Autodesk Inventor part; units mm, degrees
(part 2 of 3)
  arc A210 (178.5525, 106.028) -> (178.9163, 106.0781) centre (178.3589, 108.7773) ccw projected
  arc A211 (178.9163, 106.0781) -> (180.1512, 106.4453) centre (177.3875, 113.4813) ccw projected
  arc A212 (180.1512, 106.4453) -> (182.401, 107.5925) centre (175.3987, 118.5446) ccw projected
  arc A213 (182.401, 107.5925) -> (182.2553, 109.0714) centre (148.5, 105.0002) ccw projected
  arc A214 (182.2553, 109.0714) -> (179.825, 109.7577) centre (177.5242, 96.9636) ccw projected
  arc A215 (179.825, 109.7577) -> (178.5421, 109.8768) centre (178.487, 102.3176) ccw projected
  arc A216 (178.5421, 109.8768) -> (178.1756, 109.855) centre (178.522, 107.1208) ccw projected
  line L54 (178.1756, 109.855) -> (177.6129, 109.763) projected
  arc A217 (177.6129, 109.763) -> (177.2195, 111.7409) centre (148.5, 105.0002) ccw projected
  line L55 (177.2195, 111.7409) -> (177.7745, 111.8712) projected
  arc A218 (177.7745, 111.8712) -> (178.1215, 111.9914) centre (177.0483, 114.5299) ccw projected
  arc A219 (178.1215, 111.9914) -> (179.2611, 112.5923) centre (175.1778, 118.9541) ccw projected
  arc A220 (179.2611, 112.5923) -> (181.2438, 114.1565) centre (172.2395, 123.5321) ccw projected
  arc A221 (181.2438, 114.1565) -> (180.8125, 115.5785) centre (148.5, 105.0002) ccw projected
  arc A222 (180.8125, 115.5785) -> (178.2949, 115.7775) centre (178.5344, 102.7804) ccw projected
  arc A223 (178.2949, 115.7775) -> (177.0135, 115.644) centre (178.4342, 108.2194) ccw projected
  arc A224 (177.0135, 115.644) -> (176.6582, 115.5512) centre (177.5315, 112.937) ccw projected
  line L56 (176.6582, 115.5512) -> (176.1244, 115.3511) projected
  arc A225 (176.1244, 115.3511) -> (175.3526, 117.2143) centre (148.5, 105.0002) ccw projected
  line L57 (175.3526, 117.2143) -> (175.8716, 117.4504) projected
  arc A226 (175.8716, 117.4504) -> (176.1884, 117.6359) centre (174.6406, 119.9163) ccw projected
  arc A227 (176.1884, 117.6359) -> (177.1889, 118.4477) centre (171.943, 123.8905) ccw projected
  arc A228 (177.1889, 118.4477) -> (178.8284, 120.3685) centre (168.1679, 127.8073) ccw projected
  arc A229 (178.8284, 120.3685) -> (178.1279, 121.6791) centre (148.5, 105.0002) ccw projected
  arc A230 (178.1279, 121.6791) -> (175.6199, 121.3831) centre (178.3903, 108.6825) ccw projected
  arc A231 (175.6199, 121.3831) -> (174.3891, 121.0022) centre (177.231, 113.9974) ccw projected
  arc A232 (174.3891, 121.0022) -> (174.0588, 120.8418) centre (175.4252, 118.4483) ccw projected
  line L58 (174.0588, 120.8418) -> (173.5742, 120.5415) projected
  arc A233 (173.5742, 120.5415) -> (172.4538, 122.2183) centre (148.5, 105.0002) ccw projected
  line L59 (172.4538, 122.2183) -> (172.9167, 122.5511) projected
  arc A234 (172.9167, 122.5511) -> (173.1913, 122.7949) centre (171.2283, 124.7295) ccw projected
  arc A235 (173.1913, 122.7949) -> (174.0142, 123.7862) centre (167.8072, 128.1011) ccw projected
  arc A236 (174.0142, 123.7862) -> (175.2474, 125.99) centre (163.3405, 131.2061) ccw projected
  arc A237 (175.2474, 125.99) -> (174.3047, 127.1387) centre (148.5, 105.0002) ccw projected
  arc A238 (174.3047, 127.1387) -> (171.9026, 126.3591) centre (177.0976, 114.4431) ccw projected
  arc A239 (171.9026, 126.3591) -> (170.7698, 125.7455) centre (174.9236, 119.4296) ccw projected
  arc A240 (170.7698, 125.7455) -> (170.4771, 125.5237) centre (172.2843, 123.4427) ccw projected
  line L60 (170.4771, 125.5237) -> (170.0604, 125.1346) projected
  arc A241 (170.0604, 125.1346) -> (168.6344, 126.5606) centre (148.5, 105.0002) ccw projected
  line L61 (168.6344, 126.5606) -> (169.0235, 126.9773) projected
  arc A242 (169.0235, 126.9773) -> (169.2453, 127.27) centre (166.9426, 128.7845) ccw projected
  arc A243 (169.2453, 127.27) -> (169.8589, 128.4028) centre (162.9294, 131.4238) ccw projected
  arc A244 (169.8589, 128.4028) -> (170.6385, 130.8049) centre (157.9429, 133.5978) ccw projected
  arc A245 (170.6385, 130.8049) -> (169.4898, 131.7476) centre (148.5, 105.0002) ccw projected
  arc A246 (169.4898, 131.7476) -> (167.286, 130.5144) centre (174.7059, 119.8407) ccw projected
  arc A247 (167.286, 130.5144) -> (166.2947, 129.6915) centre (171.6009, 124.3074) ccw projected
  arc A248 (166.2947, 129.6915) -> (166.0509, 129.4169) centre (168.2293, 127.7285) ccw projected
  line L62 (166.0509, 129.4169) -> (165.7181, 128.954) projected
  arc A249 (165.7181, 128.954) -> (164.0413, 130.0744) centre (148.5, 105.0002) ccw projected
  line L63 (164.0413, 130.0744) -> (164.3416, 130.559) projected
  arc A250 (164.3416, 130.559) -> (164.502, 130.8893) centre (161.9481, 131.9254) ccw projected
  arc A251 (164.502, 130.8893) -> (164.8829, 132.1201) centre (157.4972, 133.7312) ccw projected
  arc A252 (164.8829, 132.1201) -> (165.1789, 134.6281) centre (152.1823, 134.8905) ccw projected
  arc A253 (165.1789, 134.6281) -> (163.8683, 135.3286) centre (148.5, 105.0002) ccw projected
  arc A254 (163.8683, 135.3286) -> (161.9475, 133.6891) centre (171.3071, 124.6681) ccw projected
  arc A255 (161.9475, 133.6891) -> (161.1357, 132.6886) centre (167.3903, 128.4432) ccw projected
  circle A256 centre (148.5, 105.0002) radius 2.995
  line L64 (196.9122, 102.2502) -> (196.9122, 107.7502) construction
  line L65 (196.9122, 107.7502) -> (201.6754, 105.0002) construction
  line L66 (201.6754, 105.0002) -> (196.9122, 102.2502) construction
  line L67 (148.5, 105.0002) -> (198.5, 105.0002) construction
  circle A257 centre (201.6754, 105.0002) radius 1.5
  circle A258 centre (196.9122, 102.2502) radius 1.5
  circle A259 centre (196.9122, 107.7502) radius 1.5
  circle A260 centre (198.5, 105.0002) radius 8.5
  line L68 (198.5, 113.5002) -> (157.4972, 113.5002)
  line L69 (198.5, 96.5002) -> (156.0023, 96.5002)
  line L70 (198.5, 105.0002) -> (209.904, 111.5843)
  line L71 (198.5, 105.0002) -> (211.1766, 97.6813)
  line L72 (198.5, 105.0002) -> (198.5, 117.6544)
  line L73 (198.5, 105.0002) -> (198.5, 93.004)
  circle A261 centre (198.5, 105.0002) radius 6
  point P0 (0, 0)
  point P1 (180.5064, 96.5002)
  point P2 (198.5, 99.0002)
  point P3 (203.6961, 102.0002)
  point P4 (205.8612, 100.7502)
  point P5 (205.8612, 109.2502)
  point P6 (203.6961, 108.0002)
  point P7 (198.5, 111.0002)
  point P8 (180.5064, 113.5002)
  dimension "d2" = 5.99
  dimension "d3" = 5.5
  dimension "d4" = 50
  dimension "d5" = 3
  dimension "d6" = 3
  dimension "d7" = 3
  dimension "d8" = 17
  dimension "d9" = 60
  dimension "d10" = 60
  dimension "d11" = 12
  constraints: 20 end point, 6 centre point, 6 coincident, 3 horizontal, 2 point on circle, 2 tangent, 1 collinear, 1 point on line, 1 vertical, 7 other
  measures "d2" diameter of A256
  measures "d3" distance of L64.end L65.end
  measures "d4" distance of L67.start L67.end
  measures "d5" diameter of A257
  measures "d6" diameter of A258
  measures "d7" diameter of A259
  measures "d8" diameter of A260
  measures "d9" angle of L70 L72
  measures "d10" angle of L73 L71
  measures "d11" diameter of A261
extrude "押し出し2" add sketch "スケッチ2" against normal blind 6 contours L68 A260 L69 A198 A199 A200 L50 A201 L51 A202 A203 A204 A205 A206 A207 A208 L52 A209 L53 A210 A211 A212 A213 A214 A215 A216 L54 A217 L55 A218 A219 A220 | L72 A261 L73 A260 | A260 L71 A261 L70 | A261 L70 L72 | L72 L73 A261 | L73 L71 A261 | A261 L71 L70
fillet "フィレット1" radius 2 4 edges at (198.5, 111.0002, 3) (203.6961, 108.0002, 3) (203.6961, 102.0002, 3) (198.5, 99.0002, 3)
extrude "押し出し3" cut sketch "スケッチ2" against normal blind 6 contours A256
sketch "スケッチ3" plane through (0, 0, 6) normal (0, 0, 1) x (1, 0, 0)
  circle A0 centre (148.5, 105.0002) radius 2.995 projected
  circle A1 centre (201.6754, 105.0002) radius 1.5 projected
  circle A2 centre (196.9122, 107.7502) radius 1.5 projected
  circle A3 centre (196.9122, 102.2502) radius 1.5 projected
  arc A4 (161.1357, 132.6886) -> (160.9502, 132.3718) centre (163.4161, 131.1408) ccw projected
  line L0 (160.9502, 132.3718) -> (160.7141, 131.8528) projected
  arc A5 (160.7141, 131.8528) -> (158.8509, 132.6246) centre (148.5, 105.0002) ccw projected
  line L1 (158.8509, 132.6246) -> (159.051, 133.1584) projected
  arc A6 (159.051, 133.1584) -> (159.1439, 133.5137) centre (156.4368, 134.0317) ccw projected
  arc A7 (159.1439, 133.5137) -> (159.2773, 134.7951) centre (151.7192, 134.9344) ccw projected
  arc A8 (159.2773, 134.7951) -> (159.0783, 137.3127) centre (146.2802, 135.0346) ccw projected
  arc A9 (159.0783, 137.3127) -> (157.6563, 137.744) centre (148.5, 105.0002) ccw projected
  arc A10 (157.6563, 137.744) -> (156.0922, 135.7613) centre (167.0319, 128.7396) ccw projected
  arc A11 (156.0922, 135.7613) -> (155.4912, 134.6217) centre (162.4539, 131.678) ccw projected
  arc A12 (155.4912, 134.6217) -> (155.371, 134.2747) centre (158.0297, 133.5485) ccw projected
  line L2 (155.371, 134.2747) -> (155.2407, 133.7197) projected
  arc A13 (155.2407, 133.7197) -> (153.2628, 134.1131) centre (148.5, 105.0002) ccw projected
  line L3 (153.2628, 134.1131) -> (153.3548, 134.6758) projected
  arc A14 (153.3548, 134.6758) -> (153.3766, 135.0423) centre (150.6206, 135.0222) ccw projected
  arc A15 (153.3766, 135.0423) -> (153.2575, 136.3252) centre (145.8174, 134.9872) ccw projected
  arc A16 (153.2575, 136.3252) -> (152.5712, 138.7555) centre (140.4634, 134.0244) ccw projected
  arc A17 (152.5712, 138.7555) -> (151.0923, 138.9012) centre (148.5, 105.0002) ccw projected
  arc A18 (151.0923, 138.9012) -> (149.9451, 136.6514) centre (162.0444, 131.8989) ccw projected
  arc A19 (149.9451, 136.6514) -> (149.5779, 135.4165) centre (156.9811, 133.8877) ccw projected
  arc A20 (149.5779, 135.4165) -> (149.5278, 135.0527) centre (152.2771, 134.8591) ccw projected
  line L4 (149.5278, 135.0527) -> (149.5083, 134.4829) projected
  arc A21 (149.5083, 134.4829) -> (147.4916, 134.4829) centre (148.5, 105.0002) ccw projected
  line L5 (147.4916, 134.4829) -> (147.4721, 135.0527) projected
  arc A22 (147.4721, 135.0527) -> (147.422, 135.4165) centre (144.7228, 134.8591) ccw projected
  arc A23 (147.422, 135.4165) -> (147.0549, 136.6514) centre (140.0188, 133.8877) ccw projected
  arc A24 (147.0549, 136.6514) -> (145.9076, 138.9012) centre (134.9555, 131.8989) ccw projected
  arc A25 (145.9076, 138.9012) -> (144.4287, 138.7555) centre (148.5, 105.0002) ccw projected
  arc A26 (144.4287, 138.7555) -> (143.7424, 136.3252) centre (156.5365, 134.0244) ccw projected
  arc A27 (143.7424, 136.3252) -> (143.6233, 135.0423) centre (151.1825, 134.9872) ccw projected
  arc A28 (143.6233, 135.0423) -> (143.6451, 134.6758) centre (146.3794, 135.0222) ccw projected
  line L6 (143.6451, 134.6758) -> (143.7371, 134.1131) projected
  arc A29 (143.7371, 134.1131) -> (141.7592, 133.7197) centre (148.5, 105.0002) ccw projected
  line L7 (141.7592, 133.7197) -> (141.6289, 134.2747) projected
  arc A30 (141.6289, 134.2747) -> (141.5088, 134.6217) centre (138.9702, 133.5485) ccw projected
  arc A31 (141.5088, 134.6217) -> (140.9078, 135.7613) centre (134.5461, 131.678) ccw projected
  arc A32 (140.9078, 135.7613) -> (139.3437, 137.744) centre (129.9681, 128.7396) ccw projected
  arc A33 (139.3437, 137.744) -> (137.9216, 137.3127) centre (148.5, 105.0002) ccw projected
  arc A34 (137.9216, 137.3127) -> (137.7227, 134.7951) centre (150.7197, 135.0346) ccw projected
  arc A35 (137.7227, 134.7951) -> (137.8561, 133.5137) centre (145.2808, 134.9344) ccw projected
  arc A36 (137.8561, 133.5137) -> (137.949, 133.1584) centre (140.5631, 134.0317) ccw projected
  line L8 (137.949, 133.1584) -> (138.149, 132.6246) projected
  arc A37 (138.149, 132.6246) -> (136.2858, 131.8528) centre (148.5, 105.0002) ccw projected
  line L9 (136.2858, 131.8528) -> (136.0497, 132.3718) projected
  arc A38 (136.0497, 132.3718) -> (135.8642, 132.6886) centre (133.5838, 131.1408) ccw projected
  arc A39 (135.8642, 132.6886) -> (135.0525, 133.6891) centre (129.6096, 128.4432) ccw projected
  arc A40 (135.0525, 133.6891) -> (133.1316, 135.3286) centre (125.6928, 124.6681) ccw projected
  arc A41 (133.1316, 135.3286) -> (131.821, 134.6281) centre (148.5, 105.0002) ccw projected
  arc A42 (131.821, 134.6281) -> (132.117, 132.1201) centre (144.8176, 134.8905) ccw projected
  arc A43 (132.117, 132.1201) -> (132.4979, 130.8893) centre (139.5027, 133.7312) ccw projected
  arc A44 (132.4979, 130.8893) -> (132.6583, 130.559) centre (135.0518, 131.9254) ccw projected
  line L10 (132.6583, 130.559) -> (132.9586, 130.0744) projected
  arc A45 (132.9586, 130.0744) -> (131.2818, 128.954) centre (148.5, 105.0002) ccw projected
  line L11 (131.2818, 128.954) -> (130.949, 129.4169) projected
  arc A46 (130.949, 129.4169) -> (130.7053, 129.6915) centre (128.7706, 127.7285) ccw projected
  arc A47 (130.7053, 129.6915) -> (129.7139, 130.5144) centre (125.3991, 124.3074) ccw projected
  arc A48 (129.7139, 130.5144) -> (127.5101, 131.7476) centre (122.294, 119.8407) ccw projected
  arc A49 (127.5101, 131.7476) -> (126.3614, 130.8049) centre (148.5, 105.0002) ccw projected
  arc A50 (126.3614, 130.8049) -> (127.141, 128.4028) centre (139.0571, 133.5978) ccw projected
  arc A51 (127.141, 128.4028) -> (127.7546, 127.27) centre (134.0705, 131.4238) ccw projected
  arc A52 (127.7546, 127.27) -> (127.9764, 126.9773) centre (130.0574, 128.7845) ccw projected
  line L12 (127.9764, 126.9773) -> (128.3655, 126.5606) projected
  arc A53 (128.3655, 126.5606) -> (126.9395, 125.1346) centre (148.5, 105.0002) ccw projected
  line L13 (126.9395, 125.1346) -> (126.5228, 125.5237) projected
  arc A54 (126.5228, 125.5237) -> (126.2301, 125.7455) centre (124.7157, 123.4427) ccw projected
  arc A55 (126.2301, 125.7455) -> (125.0973, 126.3591) centre (122.0763, 119.4296) ccw projected
  arc A56 (125.0973, 126.3591) -> (122.6952, 127.1387) centre (119.9023, 114.4431) ccw projected
  arc A57 (122.6952, 127.1387) -> (121.7525, 125.99) centre (148.5, 105.0002) ccw projected
  arc A58 (121.7525, 125.99) -> (122.9858, 123.7862) centre (133.6594, 131.2061) ccw projected
  arc A59 (122.9858, 123.7862) -> (123.8086, 122.7949) centre (129.1927, 128.1011) ccw projected
  arc A60 (123.8086, 122.7949) -> (124.0832, 122.5511) centre (125.7717, 124.7295) ccw projected
  line L14 (124.0832, 122.5511) -> (124.5462, 122.2183) projected
  arc A61 (124.5462, 122.2183) -> (123.4257, 120.5415) centre (148.5, 105.0002) ccw projected
  line L15 (123.4257, 120.5415) -> (122.9411, 120.8418) projected
  arc A62 (122.9411, 120.8418) -> (122.6108, 121.0022) centre (121.5747, 118.4483) ccw projected
  arc A63 (122.6108, 121.0022) -> (121.3801, 121.3831) centre (119.769, 113.9974) ccw projected
  arc A64 (121.3801, 121.3831) -> (118.8721, 121.6791) centre (118.6096, 108.6825) ccw projected
  arc A65 (118.8721, 121.6791) -> (118.1715, 120.3685) centre (148.5, 105.0002) ccw projected
  arc A66 (118.1715, 120.3685) -> (119.811, 118.4477) centre (128.832, 127.8073) ccw projected
  arc A67 (119.811, 118.4477) -> (120.8115, 117.6359) centre (125.057, 123.8905) ccw projected
  arc A68 (120.8115, 117.6359) -> (121.1284, 117.4504) centre (122.3594, 119.9163) ccw projected
  line L16 (121.1284, 117.4504) -> (121.6473, 117.2143) projected
  arc A69 (121.6473, 117.2143) -> (120.8756, 115.3511) centre (148.5, 105.0002) ccw projected
  line L17 (120.8756, 115.3511) -> (120.3417, 115.5512) projected
  arc A70 (120.3417, 115.5512) -> (119.9864, 115.644) centre (119.4685, 112.937) ccw projected
  arc A71 (119.9864, 115.644) -> (118.705, 115.7775) centre (118.5657, 108.2194) ccw projected
  arc A72 (118.705, 115.7775) -> (116.1874, 115.5785) centre (118.4655, 102.7804) ccw projected
  arc A73 (116.1874, 115.5785) -> (115.7561, 114.1565) centre (148.5, 105.0002) ccw projected
  arc A74 (115.7561, 114.1565) -> (117.7388, 112.5923) centre (124.7605, 123.5321) ccw projected
  arc A75 (117.7388, 112.5923) -> (118.8784, 111.9914) centre (121.8221, 118.9541) ccw projected
  arc A76 (118.8784, 111.9914) -> (119.2254, 111.8712) centre (119.9517, 114.5299) ccw projected
  line L18 (119.2254, 111.8712) -> (119.7804, 111.7409) projected
  arc A77 (119.7804, 111.7409) -> (119.387, 109.763) centre (148.5, 105.0002) ccw projected
  line L19 (119.387, 109.763) -> (118.8243, 109.855) projected
  arc A78 (118.8243, 109.855) -> (118.4578, 109.8768) centre (118.4779, 107.1208) ccw projected
  arc A79 (118.4578, 109.8768) -> (117.175, 109.7577) centre (118.5129, 102.3176) ccw projected
  arc A80 (117.175, 109.7577) -> (114.7446, 109.0714) centre (119.4757, 96.9636) ccw projected
  arc A81 (114.7446, 109.0714) -> (114.5989, 107.5925) centre (148.5, 105.0002) ccw projected
  arc A82 (114.5989, 107.5925) -> (116.8487, 106.4453) centre (121.6012, 118.5446) ccw projected
  arc A83 (116.8487, 106.4453) -> (118.0837, 106.0781) centre (119.6124, 113.4813) ccw projected
  arc A84 (118.0837, 106.0781) -> (118.4474, 106.028) centre (118.641, 108.7773) ccw projected
  line L20 (118.4474, 106.028) -> (119.0172, 106.0085) projected
  arc A85 (119.0172, 106.0085) -> (119.0172, 103.9918) centre (148.5, 105.0002) ccw projected
  line L21 (119.0172, 103.9918) -> (118.4474, 103.9723) projected
  arc A86 (118.4474, 103.9723) -> (118.0837, 103.9222) centre (118.641, 101.223) ccw projected
  arc A87 (118.0837, 103.9222) -> (116.8487, 103.5551) centre (119.6124, 96.519) ccw projected
  arc A88 (116.8487, 103.5551) -> (114.5989, 102.4078) centre (121.6012, 91.4557) ccw projected
  arc A89 (114.5989, 102.4078) -> (114.7446, 100.9289) centre (148.5, 105.0002) ccw projected
  arc A90 (114.7446, 100.9289) -> (117.175, 100.2426) centre (119.4757, 113.0367) ccw projected
  arc A91 (117.175, 100.2426) -> (118.4578, 100.1235) centre (118.5129, 107.6827) ccw projected
  arc A92 (118.4578, 100.1235) -> (118.8243, 100.1453) centre (118.4779, 102.8796) ccw projected
  line L22 (118.8243, 100.1453) -> (119.387, 100.2373) projected
  arc A93 (119.387, 100.2373) -> (119.7804, 98.2594) centre (148.5, 105.0002) ccw projected
  line L23 (119.7804, 98.2594) -> (119.2254, 98.1291) projected
  arc A94 (119.2254, 98.1291) -> (118.8784, 98.009) centre (119.9517, 95.4704) ccw projected
  arc A95 (118.8784, 98.009) -> (117.7388, 97.408) centre (121.8221, 91.0463) ccw projected
  arc A96 (117.7388, 97.408) -> (115.7561, 95.8439) centre (124.7605, 86.4683) ccw projected
  arc A97 (115.7561, 95.8439) -> (116.1874, 94.4218) centre (148.5, 105.0002) ccw projected
  arc A98 (116.1874, 94.4218) -> (118.705, 94.2229) centre (118.4655, 107.2199) ccw projected
  arc A99 (118.705, 94.2229) -> (119.9864, 94.3563) centre (118.5657, 101.781) ccw projected
  arc A100 (119.9864, 94.3563) -> (120.3417, 94.4491) centre (119.4685, 97.0633) ccw projected
  line L24 (120.3417, 94.4491) -> (120.8756, 94.6492) projected
  arc A101 (120.8756, 94.6492) -> (121.6473, 92.786) centre (148.5, 105.0002) ccw projected
  line L25 (121.6473, 92.786) -> (121.1284, 92.5499) projected
  arc A102 (121.1284, 92.5499) -> (120.8115, 92.3644) centre (122.3594, 90.084) ccw projected
  arc A103 (120.8115, 92.3644) -> (119.811, 91.5526) centre (125.057, 86.1098) ccw projected
  arc A104 (119.811, 91.5526) -> (118.1715, 89.6318) centre (128.832, 82.193) ccw projected
  arc A105 (118.1715, 89.6318) -> (118.8721, 88.3212) centre (148.5, 105.0002) ccw projected
  arc A106 (118.8721, 88.3212) -> (121.3801, 88.6172) centre (118.6096, 101.3178) ccw projected
  arc A107 (121.3801, 88.6172) -> (122.6108, 88.9981) centre (119.769, 96.0029) ccw projected
  arc A108 (122.6108, 88.9981) -> (122.9411, 89.1585) centre (121.5747, 91.552) ccw projected
  line L26 (122.9411, 89.1585) -> (123.4257, 89.4588) projected
  arc A109 (123.4257, 89.4588) -> (124.5462, 87.782) centre (148.5, 105.0002) ccw projected
  line L27 (124.5462, 87.782) -> (124.0832, 87.4492) projected
  arc A110 (124.0832, 87.4492) -> (123.8086, 87.2055) centre (125.7717, 85.2708) ccw projected
  arc A111 (123.8086, 87.2055) -> (122.9858, 86.2141) centre (129.1927, 81.8993) ccw projected
  arc A112 (122.9858, 86.2141) -> (121.7525, 84.0103) centre (133.6594, 78.7942) ccw projected
  arc A113 (121.7525, 84.0103) -> (122.6952, 82.8616) centre (148.5, 105.0002) ccw projected
  arc A114 (122.6952, 82.8616) -> (125.0973, 83.6412) centre (119.9023, 95.5573) ccw projected
  arc A115 (125.0973, 83.6412) -> (126.2301, 84.2548) centre (122.0763, 90.5707) ccw projected
  arc A116 (126.2301, 84.2548) -> (126.5228, 84.4766) centre (124.7157, 86.5576) ccw projected
  line L28 (126.5228, 84.4766) -> (126.9395, 84.8657) projected
  arc A117 (126.9395, 84.8657) -> (128.3655, 83.4397) centre (148.5, 105.0002) ccw projected
  line L29 (128.3655, 83.4397) -> (127.9764, 83.023) projected
  arc A118 (127.9764, 83.023) -> (127.7546, 82.7303) centre (130.0574, 81.2159) ccw projected
  arc A119 (127.7546, 82.7303) -> (127.141, 81.5975) centre (134.0705, 78.5765) ccw projected
  arc A120 (127.141, 81.5975) -> (126.3614, 79.1954) centre (139.0571, 76.4025) ccw projected
  arc A121 (126.3614, 79.1954) -> (127.5101, 78.2527) centre (148.5, 105.0002) ccw projected
  arc A122 (127.5101, 78.2527) -> (129.7139, 79.486) centre (122.294, 90.1596) ccw projected
  arc A123 (129.7139, 79.486) -> (130.7053, 80.3088) centre (125.3991, 85.6929) ccw projected
  arc A124 (130.7053, 80.3088) -> (130.949, 80.5834) centre (128.7706, 82.2718) ccw projected
  line L30 (130.949, 80.5834) -> (131.2818, 81.0464) projected
  arc A125 (131.2818, 81.0464) -> (132.9586, 79.9259) centre (148.5, 105.0002) ccw projected
  line L31 (132.9586, 79.9259) -> (132.6583, 79.4413) projected
  arc A126 (132.6583, 79.4413) -> (132.4979, 79.111) centre (135.0518, 78.0749) ccw projected
  arc A127 (132.4979, 79.111) -> (132.117, 77.8803) centre (139.5027, 76.2692) ccw projected
  arc A128 (132.117, 77.8803) -> (131.821, 75.3722) centre (144.8176, 75.1098) ccw projected
  arc A129 (131.821, 75.3722) -> (133.1316, 74.6717) centre (148.5, 105.0002) ccw projected
  arc A130 (133.1316, 74.6717) -> (135.0525, 76.3112) centre (125.6928, 85.3322) ccw projected
  arc A131 (135.0525, 76.3112) -> (135.8642, 77.3117) centre (129.6096, 81.5572) ccw projected
  arc A132 (135.8642, 77.3117) -> (136.0497, 77.6286) centre (133.5838, 78.8596) ccw projected
  line L32 (136.0497, 77.6286) -> (136.2858, 78.1475) projected
  arc A133 (136.2858, 78.1475) -> (138.149, 77.3758) centre (148.5, 105.0002) ccw projected
  line L33 (138.149, 77.3758) -> (137.949, 76.8419) projected
  arc A134 (137.949, 76.8419) -> (137.8561, 76.4866) centre (140.5631, 75.9687) ccw projected
  arc A135 (137.8561, 76.4866) -> (137.7227, 75.2052) centre (145.2808, 75.0659) ccw projected
  arc A136 (137.7227, 75.2052) -> (137.9216, 72.6876) centre (150.7197, 74.9657) ccw projected
  arc A137 (137.9216, 72.6876) -> (139.3437, 72.2563) centre (148.5, 105.0002) ccw projected
  arc A138 (139.3437, 72.2563) -> (140.9078, 74.239) centre (129.9681, 81.2607) ccw projected
  arc A139 (140.9078, 74.239) -> (141.5088, 75.3786) centre (134.5461, 78.3223) ccw projected
  arc A140 (141.5088, 75.3786) -> (141.6289, 75.7256) centre (138.9702, 76.4519) ccw projected
  line L34 (141.6289, 75.7256) -> (141.7592, 76.2806) projected
  arc A141 (141.7592, 76.2806) -> (143.7371, 75.8872) centre (148.5, 105.0002) ccw projected
  line L35 (143.7371, 75.8872) -> (143.6451, 75.3245) projected
  arc A142 (143.6451, 75.3245) -> (143.6233, 74.958) centre (146.3794, 74.9781) ccw projected
  arc A143 (143.6233, 74.958) -> (143.7424, 73.6752) centre (151.1825, 75.0131) ccw projected
  arc A144 (143.7424, 73.6752) -> (144.4287, 71.2448) centre (156.5365, 75.9759) ccw projected
  arc A145 (144.4287, 71.2448) -> (145.9076, 71.0991) centre (148.5, 105.0002) ccw projected
  arc A146 (145.9076, 71.0991) -> (147.0549, 73.3489) centre (134.9555, 78.1014) ccw projected
  arc A147 (147.0549, 73.3489) -> (147.422, 74.5839) centre (140.0188, 76.1126) ccw projected
  arc A148 (147.422, 74.5839) -> (147.4721, 74.9476) centre (144.7228, 75.1412) ccw projected
  line L36 (147.4721, 74.9476) -> (147.4916, 75.5174) projected
  arc A149 (147.4916, 75.5174) -> (149.5083, 75.5174) centre (148.5, 105.0002) ccw projected
  line L37 (149.5083, 75.5174) -> (149.5278, 74.9476) projected
  arc A150 (149.5278, 74.9476) -> (149.5779, 74.5839) centre (152.2771, 75.1412) ccw projected
  arc A151 (149.5779, 74.5839) -> (149.9451, 73.3489) centre (156.9811, 76.1126) ccw projected
  arc A152 (149.9451, 73.3489) -> (151.0923, 71.0991) centre (162.0444, 78.1014) ccw projected
  arc A153 (151.0923, 71.0991) -> (152.5712, 71.2448) centre (148.5, 105.0002) ccw projected
  arc A154 (152.5712, 71.2448) -> (153.2575, 73.6752) centre (140.4634, 75.9759) ccw projected
  arc A155 (153.2575, 73.6752) -> (153.3766, 74.958) centre (145.8174, 75.0131) ccw projected
  arc A156 (153.3766, 74.958) -> (153.3548, 75.3245) centre (150.6206, 74.9781) ccw projected
  line L38 (153.3548, 75.3245) -> (153.2628, 75.8872) projected
  arc A157 (153.2628, 75.8872) -> (155.2407, 76.2806) centre (148.5, 105.0002) ccw projected
  line L39 (155.2407, 76.2806) -> (155.371, 75.7256) projected
  arc A158 (155.371, 75.7256) -> (155.4912, 75.3786) centre (158.0297, 76.4519) ccw projected
  arc A159 (155.4912, 75.3786) -> (156.0922, 74.239) centre (162.4539, 78.3223) ccw projected
  arc A160 (156.0922, 74.239) -> (157.6563, 72.2563) centre (167.0319, 81.2607) ccw projected
  arc A161 (157.6563, 72.2563) -> (159.0783, 72.6876) centre (148.5, 105.0002) ccw projected
  arc A162 (159.0783, 72.6876) -> (159.2773, 75.2052) centre (146.2802, 74.9657) ccw projected
  arc A163 (159.2773, 75.2052) -> (159.1439, 76.4866) centre (151.7192, 75.0659) ccw projected
  arc A164 (159.1439, 76.4866) -> (159.051, 76.8419) centre (156.4368, 75.9687) ccw projected
  line L40 (159.051, 76.8419) -> (158.8509, 77.3758) projected
  arc A165 (158.8509, 77.3758) -> (160.7141, 78.1475) centre (148.5, 105.0002) ccw projected
  line L41 (160.7141, 78.1475) -> (160.9502, 77.6286) projected
  arc A166 (160.9502, 77.6286) -> (161.1357, 77.3117) centre (163.4161, 78.8596) ccw projected
  arc A167 (161.1357, 77.3117) -> (161.9475, 76.3112) centre (167.3903, 81.5572) ccw projected
  arc A168 (161.9475, 76.3112) -> (163.8683, 74.6717) centre (171.3071, 85.3322) ccw projected
  arc A169 (163.8683, 74.6717) -> (165.1789, 75.3722) centre (148.5, 105.0002) ccw projected
  arc A170 (165.1789, 75.3722) -> (164.8829, 77.8803) centre (152.1823, 75.1098) ccw projected
  arc A171 (164.8829, 77.8803) -> (164.502, 79.111) centre (157.4972, 76.2692) ccw projected
  arc A172 (164.502, 79.111) -> (164.3416, 79.4413) centre (161.9481, 78.0749) ccw projected
  line L42 (164.3416, 79.4413) -> (164.0413, 79.9259) projected
  arc A173 (164.0413, 79.9259) -> (165.7181, 81.0464) centre (148.5, 105.0002) ccw projected
  line L43 (165.7181, 81.0464) -> (166.0509, 80.5834) projected
  arc A174 (166.0509, 80.5834) -> (166.2947, 80.3088) centre (168.2293, 82.2718) ccw projected
  arc A175 (166.2947, 80.3088) -> (167.286, 79.486) centre (171.6009, 85.6929) ccw projected
  arc A176 (167.286, 79.486) -> (169.4898, 78.2527) centre (174.7059, 90.1596) ccw projected
  arc A177 (169.4898, 78.2527) -> (170.6385, 79.1954) centre (148.5, 105.0002) ccw projected
  arc A178 (170.6385, 79.1954) -> (169.8589, 81.5975) centre (157.9429, 76.4025) ccw projected
  arc A179 (169.8589, 81.5975) -> (169.2453, 82.7303) centre (162.9294, 78.5765) ccw projected
  arc A180 (169.2453, 82.7303) -> (169.0235, 83.023) centre (166.9426, 81.2159) ccw projected
  line L44 (169.0235, 83.023) -> (168.6344, 83.4397) projected
  arc A181 (168.6344, 83.4397) -> (170.0604, 84.8657) centre (148.5, 105.0002) ccw projected
  line L45 (170.0604, 84.8657) -> (170.4771, 84.4766) projected
  arc A182 (170.4771, 84.4766) -> (170.7698, 84.2548) centre (172.2843, 86.5576) ccw projected
  arc A183 (170.7698, 84.2548) -> (171.9026, 83.6412) centre (174.9236, 90.5707) ccw projected
  arc A184 (171.9026, 83.6412) -> (174.3047, 82.8616) centre (177.0976, 95.5573) ccw projected
  arc A185 (174.3047, 82.8616) -> (175.2474, 84.0103) centre (148.5, 105.0002) ccw projected
  arc A186 (175.2474, 84.0103) -> (174.0142, 86.2141) centre (163.3405, 78.7942) ccw projected
  arc A187 (174.0142, 86.2141) -> (173.1913, 87.2055) centre (167.8072, 81.8993) ccw projected
  arc A188 (173.1913, 87.2055) -> (172.9167, 87.4492) centre (171.2283, 85.2708) ccw projected
  line L46 (172.9167, 87.4492) -> (172.4538, 87.782) projected
  arc A189 (172.4538, 87.782) -> (173.5742, 89.4588) centre (148.5, 105.0002) ccw projected
  line L47 (173.5742, 89.4588) -> (174.0588, 89.1585) projected
  arc A190 (174.0588, 89.1585) -> (174.3891, 88.9981) centre (175.4252, 91.552) ccw projected
  arc A191 (174.3891, 88.9981) -> (175.6199, 88.6172) centre (177.231, 96.0029) ccw projected
  arc A192 (175.6199, 88.6172) -> (178.1279, 88.3212) centre (178.3903, 101.3178) ccw projected
  arc A193 (178.1279, 88.3212) -> (178.8284, 89.6318) centre (148.5, 105.0002) ccw projected
  arc A194 (178.8284, 89.6318) -> (177.1889, 91.5526) centre (168.1679, 82.193) ccw projected
  arc A195 (177.1889, 91.5526) -> (176.1884, 92.3644) centre (171.943, 86.1098) ccw projected
  arc A196 (176.1884, 92.3644) -> (175.8716, 92.5499) centre (174.6406, 90.084) ccw projected
  line L48 (175.8716, 92.5499) -> (175.3526, 92.786) projected
  arc A197 (175.3526, 92.786) -> (176.1244, 94.6492) centre (148.5, 105.0002) ccw projected
  line L49 (176.1244, 94.6492) -> (176.6582, 94.4491) projected
  arc A198 (176.6582, 94.4491) -> (177.0135, 94.3563) centre (177.5315, 97.0633) ccw projected
  arc A199 (177.0135, 94.3563) -> (178.2949, 94.2229) centre (178.4342, 101.781) ccw projected
  arc A200 (178.2949, 94.2229) -> (180.8125, 94.4218) centre (178.5344, 107.2199) ccw projected
  arc A201 (180.8125, 94.4218) -> (181.2438, 95.8439) centre (148.5, 105.0002) ccw projected
  arc A202 (181.2438, 95.8439) -> (180.5064, 96.5002) centre (172.2395, 86.4683) ccw projected
  line L50 (180.5064, 96.5002) -> (198.5, 96.5002) projected
  line L51 (198.5, 96.5002) -> (198.5, 97.2542) projected
  arc A203 (200, 99.1907) -> (198.5, 97.2542) centre (200.5, 97.2542) ccw projected
  arc A204 (200, 99.1907) -> (202.7811, 100.7964) centre (198.5, 105.0002) ccw projected
  arc A205 (205.2082, 101.1272) -> (202.7811, 100.7964) centre (204.2082, 99.3951) ccw projected
  line L52 (205.2082, 101.1272) -> (205.8612, 100.7502) projected
  arc A206 (205.8612, 100.7502) -> (205.8612, 109.2502) centre (198.5, 105.0002) ccw projected
  line L53 (205.8612, 109.2502) -> (205.2082, 108.8731) projected
  arc A207 (202.7811, 109.2039) -> (205.2082, 108.8731) centre (204.2082, 110.6052) ccw projected
  arc A208 (202.7811, 109.2039) -> (200, 110.8096) centre (198.5, 105.0002) ccw projected
  arc A209 (198.5, 112.7461) -> (200, 110.8096) centre (200.5, 112.7461) ccw projected
  line L54 (198.5, 112.7461) -> (198.5, 113.5002) projected
  line L55 (198.5, 113.5002) -> (180.5064, 113.5002) projected
  arc A210 (180.5064, 113.5002) -> (181.2438, 114.1565) centre (172.2395, 123.5321) ccw projected
  arc A211 (181.2438, 114.1565) -> (180.8125, 115.5785) centre (148.5, 105.0002) ccw projected
  arc A212 (180.8125, 115.5785) -> (178.2949, 115.7775) centre (178.5344, 102.7804) ccw projected
  arc A213 (178.2949, 115.7775) -> (177.0135, 115.644) centre (178.4342, 108.2194) ccw projected
  arc A214 (177.0135, 115.644) -> (176.6582, 115.5512) centre (177.5315, 112.937) ccw projected
  line L56 (176.6582, 115.5512) -> (176.1244, 115.3511) projected
  arc A215 (176.1244, 115.3511) -> (175.3526, 117.2143) centre (148.5, 105.0002) ccw projected
  line L57 (175.3526, 117.2143) -> (175.8716, 117.4504) projected
  arc A216 (175.8716, 117.4504) -> (176.1884, 117.6359) centre (174.6406, 119.9163) ccw projected
  arc A217 (176.1884, 117.6359) -> (177.1889, 118.4477) centre (171.943, 123.8905) ccw projected
  arc A218 (177.1889, 118.4477) -> (178.8284, 120.3685) centre (168.1679, 127.8073) ccw projected
  arc A219 (178.8284, 120.3685) -> (178.1279, 121.6791) centre (148.5, 105.0002) ccw projected
  arc A220 (178.1279, 121.6791) -> (175.6199, 121.3831) centre (178.3903, 108.6825) ccw projected
  arc A221 (175.6199, 121.3831) -> (174.3891, 121.0022) centre (177.231, 113.9974) ccw projected
  arc A222 (174.3891, 121.0022) -> (174.0588, 120.8418) centre (175.4252, 118.4483) ccw projected
  line L58 (174.0588, 120.8418) -> (173.5742, 120.5415) projected
  arc A223 (173.5742, 120.5415) -> (172.4538, 122.2183) centre (148.5, 105.0002) ccw projected
  line L59 (172.4538, 122.2183) -> (172.9167, 122.5511) projected
  arc A224 (172.9167, 122.5511) -> (173.1913, 122.7949) centre (171.2283, 124.7295) ccw projected
  arc A225 (173.1913, 122.7949) -> (174.0142, 123.7862) centre (167.8072, 128.1011) ccw projected
  arc A226 (174.0142, 123.7862) -> (175.2474, 125.99) centre (163.3405, 131.2061) ccw projected
  arc A227 (175.2474, 125.99) -> (174.3047, 127.1387) centre (148.5, 105.0002) ccw projected
  arc A228 (174.3047, 127.1387) -> (171.9026, 126.3591) centre (177.0976, 114.4431) ccw projected
  arc A229 (171.9026, 126.3591) -> (170.7698, 125.7455) centre (174.9236, 119.4296) ccw projected
  arc A230 (170.7698, 125.7455) -> (170.4771, 125.5237) centre (172.2843, 123.4427) ccw projected
  line L60 (170.4771, 125.5237) -> (170.0604, 125.1346) projected
  arc A231 (170.0604, 125.1346) -> (168.6344, 126.5606) centre (148.5, 105.0002) ccw projected
  line L61 (168.6344, 126.5606) -> (169.0235, 126.9773) projected
  arc A232 (169.0235, 126.9773) -> (169.2453, 127.27) centre (166.9426, 128.7845) ccw projected
  arc A233 (169.2453, 127.27) -> (169.8589, 128.4028) centre (162.9294, 131.4238) ccw projected
  arc A234 (169.8589, 128.4028) -> (170.6385, 130.8049) centre (157.9429, 133.5978) ccw projected
  arc A235 (170.6385, 130.8049) -> (169.4898, 131.7476) centre (148.5, 105.0002) ccw projected
  arc A236 (169.4898, 131.7476) -> (167.286, 130.5144) centre (174.7059, 119.8407) ccw projected
  arc A237 (167.286, 130.5144) -> (166.2947, 129.6915) centre (171.6009, 124.3074) ccw projected
  arc A238 (166.2947, 129.6915) -> (166.0509, 129.4169) centre (168.2293, 127.7285) ccw projected
  line L62 (166.0509, 129.4169) -> (165.7181, 128.954) projected
  arc A239 (165.7181, 128.954) -> (164.0413, 130.0744) centre (148.5, 105.0002) ccw projected
  line L63 (164.0413, 130.0744) -> (164.3416, 130.559) projected
  arc A240 (164.3416, 130.559) -> (164.502, 130.8893) centre (161.9481, 131.9254) ccw projected
  arc A241 (164.502, 130.8893) -> (164.8829, 132.1201) centre (157.4972, 133.7312) ccw projected
  arc A242 (164.8829, 132.1201) -> (165.1789, 134.6281) centre (152.1823, 134.8905) ccw projected
  arc A243 (165.1789, 134.6281) -> (163.8683, 135.3286) centre (148.5, 105.0002) ccw projected
  arc A244 (163.8683, 135.3286) -> (161.9475, 133.6891) centre (171.3071, 124.6681) ccw projected
  arc A245 (161.9475, 133.6891) -> (161.1357, 132.6886) centre (167.3903, 128.4432) ccw projected
  circle A246 centre (148.5, 105.0002) radius 24.5
  circle A247 centre (196.9122, 107.7502) radius 4.5
  circle A248 centre (196.9122, 102.2502) radius 4.5
  line L64 (193.3503, 110.5002) -> (151.9089, 110.5002)
  line L65 (193.3503, 99.5002) -> (154.3025, 99.5002)
  line L66 (148.5, 105.0002) -> (141.7592, 76.2806)
  line L67 (148.5, 105.0002) -> (164.0413, 130.0744)
  circle A249 centre (148.5, 105.0002) radius 7.995
  line L68 (180.5064, 113.5002) -> (153.7684, 113.5002)
  arc A250 (181.2438, 95.8439) -> (180.5064, 96.5002) centre (172.2395, 86.4683) ccw projected
  line L69 (180.5064, 96.5002) -> (146.5049, 96.5002)
  point P0 (0, 0)
  point P1 (150.0778, 107.5458)
  point P2 (147.8156, 102.0844)
  dimension "d17" = 5
  dimension "d18" = 3
  dimension "d19" = 3
  dimension "d20" = 3
  dimension "d21" = 3
  dimension "d22" = 5
  constraints: 12 end point, 4 horizontal, 3 point on line, 1 centre point, 1 coincident, 9 other
  measures "d17" radial gap between concentric circles of A21 A246
  measures "d18" diameter of A2
  measures "d19" diameter of A3
  measures "d20" distance between parallel lines of L64 L55
  measures "d21" distance between parallel lines of L50 L65
extrude "押し出し4" cut sketch "スケッチ3" against normal blind 6 contours A0 L66 L67 | L69 A246 L66 | L67 A246 L68 | A246 L69 A202 A201 A200 A199 A198 L49 A197 L48 A196 A195 A194 A193 A192 A191 A190 L47 A189 L46 A188 A187 A186 A185 A184 A183 A182 L45 A181 L44 A180 A179 A178 A177 A176 A175 A174 L43 A173 L42 A172 A171 A170 A169 A168 A167 A166 L41 A165 L40 A164 A163 A162 A161 A160 A159 A158 L39 A157 L38 A156 A155 A154 A153 A152 A151 A150 L37 A149 L36 A148 A147 A146 A145 A144 A143 A142 L35 A141 L66 | A246 L67 A239 L62 A238 A237 A236 A235 A234 A233 A232 L61 A231 L60 A230 A229 A228 A227 A226 A225 A224 L59 A223 L58 A222 A221 A220 A219 A218 A217 A216 L57 A215 L56 A214 A213 A212 A211 A210 L68 | A247 A3 | A3 A247 | A248 A2 | A2 A248 | A247 A248 A1 | A1 A248 A247 | A247 A248 A1 | A1 A248 A247 picked at (149.1474, 103.1248)
fillet "フィレット3" radius 5 1 edges at (146.5049, 96.5002, 3)
fillet "フィレット3" radius 2 1 edges at (153.7684, 113.5002, 3)
sketch "スケッチ4" plane through (0, 0, 6) normal (0, 0, 1) x (1, 0, 0)
  point P0 (0, 0)